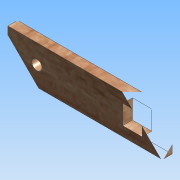
# Autodesk Inventor part: slider_box
Saved by Autodesk Inventor 2015 (Build 190159000, 159)
## iProperties
Created: 2014-09-30
Part Number: slider_box
Material: Wood (Birch)
Document SubType Name: Modeling
Designer: shohei
Density: 0.55 g/cm^3
Appearance: Birch - Natural Polished
Author: shohei
Autodesk Inventor part; units mm, degrees
ref_plane "YZ Plane" through (0, 0, 0) normal (1, 0, 0) x (0, 1, 0)
ref_plane "XZ Plane" through (0, 0, 0) normal (0, 1, 0) x (-1, 0, 0)
ref_plane "XY Plane" through (0, 0, 0) normal (0, 0, 1) x (1, 0, 0)
sketch "Sketch1" plane through (0, 0, 0) normal (0, 1, 0) x (-1, 0, 0)
  line L0 (0, 0) -> (80, 0)
  line L1 (80, 0) -> (80, 20)
  line L2 (80, 20) -> (0, 20)
  line L3 (0, 20) -> (0, 0)
  circle A0 centre (65, 10) radius 2.6
  dimension "d2" = 20
  dimension "d3" = 80
  dimension "d4" = 5.2
  dimension "d7" = 15
  dimension "d8" = 10
  constraints: 8 end point, 2 parallel, 1 centre point, 1 horizontal, 1 perpendicular
  measures "d2" distance of L0.end L1.end
  measures "d3" distance of L1.end L2.end
  measures "d4" diameter of A0
  measures "d7" distance from line of L1 A0.centre
  measures "d8" distance from line of L2 A0.centre
extrude "Extrusion2" add sketch "Sketch1" along normal blind 5
sketch "Sketch3" plane through (0, 5, 0) normal (0, 1, 0) x (1, 0, 0)
  circle A0 centre (-65, -10) radius 2.6 projected
  line L0 (0, 0) -> (-80, 0) projected
  line L1 (-80, 0) -> (-80, -20) projected
  line L2 (-80, -20) -> (0, -20) projected
  line L3 (0, -20) -> (0, 0) projected
  line L4 (-10.5, -5) -> (-20.5, -5)
  line L5 (-20.5, -5) -> (-20.5, -15)
  line L6 (-20.5, -15) -> (-10.5, -15)
  line L7 (-10.5, -15) -> (-10.5, -5)
  line L8 (-10.5, -5) -> (-20.5, -15) construction
  line L9 (-20.5, -5) -> (-10.5, -15) construction
  point P0 (-15.5, -10)
  dimension "d11" = 10
  dimension "d12" = 10
  dimension "d17" = 64.5
  dimension "d18" = 10
  constraints: 12 end point, 2 midpoint, 2 parallel, 1 horizontal, 1 perpendicular
  measures "d11" distance of L6.end L5.end
  measures "d12" distance of L5.end L4.end
  measures "d17" distance from line of point (-15.5, -10) L1
  measures "d18" distance from line of L0 point (-15.5, -10)
extrude "Extrusion3" cut sketch "Sketch3" against normal through all contours L7 L6 L5 L4
equation "\"d8\" = 0.5 * d2"
equation "\"d18\" = 0.5 * d2"
body "Solid2"
